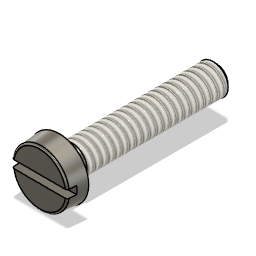
Bio Integrator (Autodesk Fusion 360 archive; units mm, degrees)
design "Vite a testa cilindrica DIN 84 - M1.6 x 8 Acciaio 4.6 Radente"
description: Vite a testa cilindrica DIN 84 - M1.6 x 8
part number: DIN 84 - M1.6 x 8 Acciaio 4.6 Radente
Autodesk Fusion 360 part; units mm, degrees
sketch "Sketch1" plane through (0, 0, 0) normal (0, 1, 0) x (1, 0, 0)
  line L0 (-0.8, 8) -> (0, 8)
  line L1 (0, 8) -> (0, -1)
  line L2 (-0.7053, 0) -> (-1.5, 0)
  line L3 (0, -1) -> (-1.4125, -1)
  line L4 (-1.4125, -1) -> (-1.5, 0)
  line L5 (-0.7053, 0) -> (-0.7053, 0.5359)
  line L6 (-0.8, 0.7) -> (-0.8, 8)
  line L7 (-0.8, 8) -> (0, 8)
  line L8 (-0.8, 0.7) -> (-0.7053, 0.5359)
  line L9 (0, -1.75) -> (0, -22.5)
  dimension "d66" = 3
  dimension "d93" = 1.4106
  dimension "d95" = 1.6
  dimension "d97" = 150
  dimension "d100" = 85
  dimension "d145" = 1
  dimension "d146" = 8
  dimension "d147" = 0.7
  constraint collinear origin L1.end L0.end
  constraint coincident origin L2
  constraint vertical L1
  constraint perpendicular L1 L3
  constraint perpendicular L2 L5
  constraint perpendicular L2 L6
  constraint perpendicular L6 L7
  constraint coincident L0.start L6.end
  constraint coincident L3.end L4.start
  measures "d97" angle of L6 L8
  measures "d100" angle of L2 L4
  measures "d145" distance of L2 L3
  measures "d146" distance of origin L7
  measures "d147" distance of L2 L6.start
revolve "Revolve1" add sketch "Sketch1" angle 360 about axis through (0, 0, -8) along (0, 0, 1)
fillet "Fillet4" radius 0.1 1 edges at (-1.3169, 0.5108, 1)
ref_plane "WorkPlane1" through (0, 0, 1) normal (0, 0, 1) x (1, 0, 0)
sketch "Sketch7" plane through (0, 0, 1) normal (0, 0, 1) x (1, 0, 0)
  line L0 (-1.5, 0.2) -> (1.5, 0.2)
  line L1 (1.5, 0.2) -> (1.5, -0.2)
  line L2 (1.5, -0.2) -> (-1.5, -0.2)
  line L3 (-1.5, -0.2) -> (-1.5, 0.2)
  line L4 (-1.5, 0) -> (1.5, 0) construction
  circle A0 centre (0, 0) radius 1.5
  dimension "d148" = 0.4
  constraint horizontal L0
  constraint vertical L1
  constraint horizontal L2
  constraint vertical L3
  constraint midpoint L3 L4.start
  constraint midpoint L1 L4.end
  constraint coincident A0.centre L4
  constraint tangent L3 A0
  constraint tangent L1 A0
  measures "d148" distance of L0 L2
extrude "Extrude3" cut sketch "Sketch7" against normal blind 0.45 contours L0 L2 A0
thread "Thread1" "ISO Metric profile 1.6 M1.6x0.35 M1.6x0.35 6g" major diameter 1.5385 minor diameter 1.1385 pitch 0.35 angle 60 resizes the face on face at (-0.796, 0.0797, -5.5667)
sketch "Sketch8" plane through (0, 0, 0) normal (0, 1, 0) x (1, 0, 0)
  line L0 (0, 8) -> (0, -1)
  line L1 (0, 8) -> (-0.816, 8)
  line L2 (-0.816, 8) -> (-0.816, 7.7853)
  line L3 (-0.816, 7.7853) -> (-0.5853, 8)
  line L4 (0, 8) -> (0, 0) construction
  dimension "d149" = 0.5853
  dimension "d150" = 0.816
  dimension "d151" = 0.2147
  constraint coincident L0.start L1.start
  constraint perpendicular L0 L1
  constraint coincident L1 L3.end
  constraint coincident L4.end origin
  measures "d149" distance of L3.end L4
  measures "d150" distance of L2 L4
  measures "d151" distance of L1 L2.end
revolve "Revolve3" cut sketch "Sketch8" angle 360 about axis through (0, 0, 1.75) along (0, 0, 1)
equation "adsk_nomlen = 8.00 mm"
equation "adsk_headh = 1.00 mm"
equation "adsk_headdia = 3.00 mm"
equation "adsk_nomdia = 1.60 mm"
equation "d66 = adsk_headdia"
equation "d71 = adsk_headh"
equation "adsk_slotdepth = 0.45 mm"
equation "adsk_slotw = 0.40 mm"
equation "d78 = -adsk_slotdepth"
equation "adsk_thrlen = 7.30 mm"
equation "adsk_headtoprad = 0.10 mm"
equation "d93 = adsk_shnkdia"
equation "d95 = adsk_nomdia"
equation "adsk_shnkdia = 1.4105569 mm"
equation "adsk_endpointdia = 1.170585 mm"
equation "adsk_startlen = 0.214707 mm"
equation "d116 = adsk_headtoprad"
equation "d145 = adsk_headh"
equation "d146 = adsk_nomlen"
equation "d147 = adsk_nomlen - adsk_thrlen"
equation "d148 = adsk_slotw"
equation "d149 = adsk_endpointdia / 2"
equation "d150 = adsk_nomdia * 0.51"
equation "d151 = adsk_startlen"

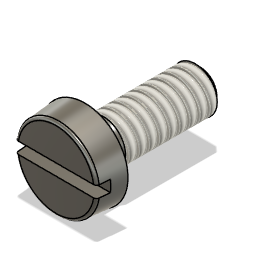
design "Vite a testa cilindrica DIN 84 - M1.6 x 4 Acciaio 4.6 Radente"
description: Vite a testa cilindrica DIN 84 - M1.6 x 4
part number: DIN 84 - M1.6 x 4 Acciaio 4.6 Radente
Autodesk Fusion 360 part; units mm, degrees
sketch "Sketch1" plane through (0, 0, 0) normal (0, 1, 0) x (1, 0, 0)
  line L0 (-0.8, 4) -> (0, 4)
  line L1 (0, 4) -> (0, -1)
  line L2 (-0.7053, 0) -> (-1.5, 0)
  line L3 (0, -1) -> (-1.4125, -1)
  line L4 (-1.4125, -1) -> (-1.5, 0)
  line L5 (-0.7053, 0) -> (-0.7053, 0.5359)
  line L6 (-0.8, 0.7) -> (-0.8, 4)
  line L7 (-0.8, 4) -> (0, 4)
  line L8 (-0.8, 0.7) -> (-0.7053, 0.5359)
  line L9 (0, -1.75) -> (0, -22.5)
  dimension "d66" = 3
  dimension "d93" = 1.4106
  dimension "d95" = 1.6
  dimension "d97" = 150
  dimension "d100" = 85
  dimension "d145" = 1
  dimension "d146" = 4
  dimension "d147" = 0.7
  constraint collinear origin L1.end L0.end
  constraint coincident origin L2
  constraint vertical L1
  constraint perpendicular L1 L3
  constraint perpendicular L2 L5
  constraint perpendicular L2 L6
  constraint perpendicular L6 L7
  constraint coincident L0.start L6.end
  constraint coincident L3.end L4.start
  measures "d97" angle of L6 L8
  measures "d100" angle of L2 L4
  measures "d145" distance of L2 L3
  measures "d146" distance of origin L7
  measures "d147" distance of L2 L6.start
revolve "Revolve1" add sketch "Sketch1" angle 360 about axis through (0, 0, -4) along (0, 0, 1)
fillet "Fillet4" radius 0.1 1 edges at (-1.3169, 0.5108, 1)
ref_plane "WorkPlane1" through (0, 0, 1) normal (0, 0, 1) x (1, 0, 0)
sketch "Sketch7" plane through (0, 0, 1) normal (0, 0, 1) x (1, 0, 0)
  line L0 (-1.5, 0.2) -> (1.5, 0.2)
  line L1 (1.5, 0.2) -> (1.5, -0.2)
  line L2 (1.5, -0.2) -> (-1.5, -0.2)
  line L3 (-1.5, -0.2) -> (-1.5, 0.2)
  line L4 (-1.5, 0) -> (1.5, 0) construction
  circle A0 centre (0, 0) radius 1.5
  dimension "d148" = 0.4
  constraint horizontal L0
  constraint vertical L1
  constraint horizontal L2
  constraint vertical L3
  constraint midpoint L3 L4.start
  constraint midpoint L1 L4.end
  constraint coincident A0.centre L4
  constraint tangent L3 A0
  constraint tangent L1 A0
  measures "d148" distance of L0 L2
extrude "Extrude3" cut sketch "Sketch7" against normal blind 0.45 contours L0 L2 A0
thread "Thread1" "ISO Metric profile 1.6 M1.6x0.35 M1.6x0.35 6g" major diameter 1.5385 minor diameter 1.1385 pitch 0.35 angle 60 resizes the face on face at (-0.799, 0.0399, -2.9)
sketch "Sketch8" plane through (0, 0, 0) normal (0, 1, 0) x (1, 0, 0)
  line L0 (0, 4) -> (0, -1)
  line L1 (0, 4) -> (-0.816, 4)
  line L2 (-0.816, 4) -> (-0.816, 3.7853)
  line L3 (-0.816, 3.7853) -> (-0.5853, 4)
  line L4 (0, 4) -> (0, 0) construction
  dimension "d149" = 0.5853
  dimension "d150" = 0.816
  dimension "d151" = 0.2147
  constraint coincident L0.start L1.start
  constraint perpendicular L0 L1
  constraint coincident L1 L3.end
  constraint coincident L4.end origin
  measures "d149" distance of L3.end L4
  measures "d150" distance of L2 L4
  measures "d151" distance of L1 L2.end
revolve "Revolve3" cut sketch "Sketch8" angle 360 about axis through (0, 0, 1.75) along (0, 0, 1)
equation "adsk_nomlen = 4.00 mm"
equation "adsk_headh = 1.00 mm"
equation "adsk_headdia = 3.00 mm"
equation "adsk_nomdia = 1.60 mm"
equation "d66 = adsk_headdia"
equation "d71 = adsk_headh"
equation "adsk_slotdepth = 0.45 mm"
equation "adsk_slotw = 0.40 mm"
equation "d78 = -adsk_slotdepth"
equation "adsk_thrlen = 3.30 mm"
equation "adsk_headtoprad = 0.10 mm"
equation "d93 = adsk_shnkdia"
equation "d95 = adsk_nomdia"
equation "adsk_shnkdia = 1.4105569 mm"
equation "adsk_endpointdia = 1.170585 mm"
equation "adsk_startlen = 0.214707 mm"
equation "d116 = adsk_headtoprad"
equation "d145 = adsk_headh"
equation "d146 = adsk_nomlen"
equation "d147 = adsk_nomlen - adsk_thrlen"
equation "d148 = adsk_slotw"
equation "d149 = adsk_endpointdia / 2"
equation "d150 = adsk_nomdia * 0.51"
equation "d151 = adsk_startlen"

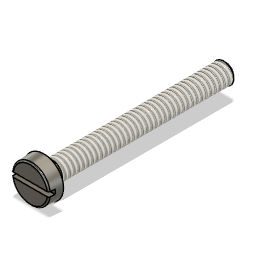
design "Vite a testa cilindrica DIN 84 - M1.4 x 12 Acciaio 4.6 Radente"
description: Vite a testa cilindrica DIN 84 - M1.4 x 12
part number: DIN 84 - M1.4 x 12 Acciaio 4.6 Radente
Autodesk Fusion 360 part; units mm, degrees
sketch "Sketch1" plane through (0, 0, 0) normal (0, 1, 0) x (1, 0, 0)
  line L0 (-0.7, 12) -> (0, 12)
  line L1 (0, 12) -> (0, -0.9)
  line L2 (-0.6188, 0) -> (-1.3, 0)
  line L3 (0, -0.9) -> (-1.2213, -0.9)
  line L4 (-1.2213, -0.9) -> (-1.3, 0)
  line L5 (-0.6188, 0) -> (-0.6188, 0.4594)
  line L6 (-0.7, 0.6) -> (-0.7, 12)
  line L7 (-0.7, 12) -> (0, 12)
  line L8 (-0.7, 0.6) -> (-0.6188, 0.4594)
  line L9 (0, -1.75) -> (0, -22.5)
  dimension "d66" = 2.6
  dimension "d93" = 1.2376
  dimension "d95" = 1.4
  dimension "d97" = 150
  dimension "d100" = 85
  dimension "d145" = 0.9
  dimension "d146" = 12
  dimension "d147" = 0.6
  constraint collinear origin L1.end L0.end
  constraint coincident origin L2
  constraint vertical L1
  constraint perpendicular L1 L3
  constraint perpendicular L2 L5
  constraint perpendicular L2 L6
  constraint perpendicular L6 L7
  constraint coincident L0.start L6.end
  constraint coincident L3.end L4.start
  measures "d97" angle of L6 L8
  measures "d100" angle of L2 L4
  measures "d145" distance of L2 L3
  measures "d146" distance of origin L7
  measures "d147" distance of L2 L6.start
revolve "Revolve1" add sketch "Sketch1" angle 360 about axis through (0, 0, -12) along (0, 0, 1)
fillet "Fillet4" radius 0.1 1 edges at (-1.1386, 0.4416, 0.9)
ref_plane "WorkPlane1" through (0, 0, 0.9) normal (0, 0, 1) x (1, 0, 0)
sketch "Sketch7" plane through (0, 0, 0.9) normal (0, 0, 1) x (1, 0, 0)
  line L0 (-1.3, 0.15) -> (1.3, 0.15)
  line L1 (1.3, 0.15) -> (1.3, -0.15)
  line L2 (1.3, -0.15) -> (-1.3, -0.15)
  line L3 (-1.3, -0.15) -> (-1.3, 0.15)
  line L4 (-1.3, 0) -> (1.3, 0) construction
  circle A0 centre (0, 0) radius 1.3
  dimension "d148" = 0.3
  constraint horizontal L0
  constraint vertical L1
  constraint horizontal L2
  constraint vertical L3
  constraint midpoint L3 L4.start
  constraint midpoint L1 L4.end
  constraint coincident A0.centre L4
  constraint tangent L3 A0
  constraint tangent L1 A0
  measures "d148" distance of L0 L2
extrude "Extrude3" cut sketch "Sketch7" against normal blind 0.4 contours L0 L2 A0
thread "Thread1" "ISO Metric profile 1.4 M1.4x0.3 M1.4x0.3 6g" major diameter 1.3455 minor diameter 1.1182 pitch 0.3 angle 60 resizes the face on face at (-0.6965, 0.0697, -8.2)
sketch "Sketch8" plane through (0, 0, 0) normal (0, 1, 0) x (1, 0, 0)
  line L0 (0, 12) -> (0, -0.9)
  line L1 (0, 12) -> (-0.714, 12)
  line L2 (-0.714, 12) -> (-0.714, 11.816)
  line L3 (-0.714, 11.816) -> (-0.516, 12)
  line L4 (0, 12) -> (0, 0) construction
  dimension "d149" = 0.516
  dimension "d150" = 0.714
  dimension "d151" = 0.184
  constraint coincident L0.start L1.start
  constraint perpendicular L0 L1
  constraint coincident L1 L3.end
  constraint coincident L4.end origin
  measures "d149" distance of L3.end L4
  measures "d150" distance of L2 L4
  measures "d151" distance of L1 L2.end
revolve "Revolve3" cut sketch "Sketch8" angle 360 about axis through (0, 0, 1.75) along (0, 0, 1)
equation "adsk_nomlen = 12.00 mm"
equation "adsk_headh = 0.90 mm"
equation "adsk_headdia = 2.60 mm"
equation "adsk_nomdia = 1.40 mm"
equation "d66 = adsk_headdia"
equation "d71 = adsk_headh"
equation "adsk_slotdepth = 0.40 mm"
equation "adsk_slotw = 0.30 mm"
equation "d78 = -adsk_slotdepth"
equation "adsk_thrlen = 11.40 mm"
equation "adsk_headtoprad = 0.10 mm"
equation "d93 = adsk_shnkdia"
equation "d95 = adsk_nomdia"
equation "adsk_shnkdia = 1.2376202 mm"
equation "adsk_endpointdia = 1.03193 mm"
equation "adsk_startlen = 0.184035 mm"
equation "d116 = adsk_headtoprad"
equation "d145 = adsk_headh"
equation "d146 = adsk_nomlen"
equation "d147 = adsk_nomlen - adsk_thrlen"
equation "d148 = adsk_slotw"
equation "d149 = adsk_endpointdia / 2"
equation "d150 = adsk_nomdia * 0.51"
equation "d151 = adsk_startlen"
